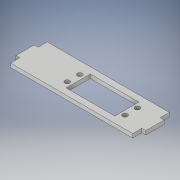
# Autodesk Inventor part: BASE_SOST.SERVO
Saved by Autodesk Inventor 2019 (Build 230136000, 136)
## iProperties
Created: 2020-02-12
Part Number: BASE_SOST.SERVO
Material: Genérico
Document SubType Name: Modeling
Designer: omar-
Density: 1 g/cm^3
Appearance: Valor por defecto
Author: omar-
Autodesk Inventor part; units mm, degrees
ref_plane "YZ Plane" through (0, 0, 0) normal (1, 0, 0) x (0, 1, 0)
ref_plane "XZ Plane" through (0, 0, 0) normal (0, 1, 0) x (-1, 0, 0)
ref_plane "XY Plane" through (0, 0, 0) normal (0, 0, 1) x (1, 0, 0)
sketch "Boceto2" plane through (0, 0, 0) normal (0, 1, 0) x (-1, 0, 0)
  circle A0 centre (0, 0) radius 5
  line L0 (9.66, 9.91) -> (-30.22, 9.91)
  line L1 (-30.22, 9.91) -> (-30.22, -9.91)
  line L2 (-30.22, -9.91) -> (9.66, -9.91)
  line L3 (9.66, -9.91) -> (9.66, 9.91)
  circle A1 centre (-33.79, 5.085) radius 2
  circle A2 centre (13.47, -5.085) radius 2
  circle A3 centre (13.47, 5.085) radius 2
  circle A4 centre (-33.79, -5.085) radius 2
  line L4 (-50, 15) -> (50, 15)
  line L5 (50, 15) -> (50, -15)
  line L6 (50, -15) -> (-50, -15)
  line L7 (-50, -15) -> (-50, 15)
  line L8 (-50, 15) -> (50, -15) construction
  line L9 (50, 15) -> (-50, -15) construction
  line L10 (53.18, 7.5) -> (50, 7.5)
  line L11 (50, 7.5) -> (50, -7.5)
  line L12 (50, -7.5) -> (53.18, -7.5)
  line L13 (53.18, -7.5) -> (53.18, 7.5)
  line L14 (-50, 7.5) -> (-53.18, 7.5)
  line L15 (-53.18, 7.5) -> (-53.18, -7.5)
  line L16 (-53.18, -7.5) -> (-50, -7.5)
  line L17 (-50, -7.5) -> (-50, 7.5)
  dimension "d2" = 10
  dimension "d3" = 9.91
  dimension "d4" = 19.82
  dimension "d5" = 9.66
  dimension "d6" = 39.88
  dimension "d7" = 4
  dimension "d8" = 4
  dimension "d9" = 4
  dimension "d10" = 5.085
  dimension "d11" = 10.17
  dimension "d12" = 13.47
  dimension "d13" = 13.47
  dimension "d14" = 4
  dimension "d15" = 33.79
  dimension "d16" = 33.79
  dimension "d17" = 5.085
  dimension "d18" = 10.17
  dimension "d19" = 100
  dimension "d20" = 30
  dimension "d21" = 3.18
  dimension "d22" = 15
  dimension "d23" = 7.5
  dimension "d24" = 15
  dimension "d25" = 3.18
  dimension "d26" = 7.5
  constraints: 36 end point, 8 parallel, 5 centre point, 4 horizontal, 4 perpendicular, 2 collinear, 2 midpoint, 1 coincident
  measures "d2" diameter of A0
  measures "d3" distance from line of L2 point (0, 0)
  measures "d4" distance of L2.end L0.start
  measures "d5" distance from line of point (0, 0) L3
  measures "d6" distance of L1.end L2.end
  measures "d7" diameter of A1
  measures "d8" diameter of A2
  measures "d9" diameter of A3
  measures "d10" vertical distance of point (0, 0) A3.centre
  measures "d11" distance of A2.centre A3.centre
  measures "d12" horizontal distance of point (0, 0) A3.centre
  measures "d13" horizontal distance of point (0, 0) A2.centre
  measures "d14" diameter of A4
  measures "d15" horizontal distance of A4.centre point (0, 0)
  measures "d16" horizontal distance of A1.centre point (0, 0)
  measures "d17" vertical distance of A4.centre point (0, 0)
  measures "d18" distance of A4.centre A1.centre
  measures "d19" distance of L5.end L6.end
  measures "d20" distance of L4.end L5.end
  measures "d21" distance of L14.start L14.end
  measures "d22" distance of L14.end L15.end
  measures "d23" distance between parallel lines of L6 L16
  measures "d24" distance of L12.end L10.start
  measures "d25" distance of L11.end L12.end
  measures "d26" distance between parallel lines of L6 L12
extrude "Extrusión1" add sketch "Boceto2" along normal blind 3.18 contours L4 L5 L6 L7 | L7 L16 L15 L14 | L10 L13 L12 L5
